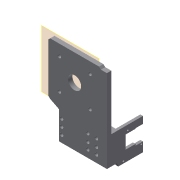
# Autodesk Inventor part: 10_Adapter_Laser_XY_left
Saved by Autodesk Inventor 2019 (Build 230136000, 136)
## iProperties
Created: 2019-05-02
Part Number: 10_Adapter_Laser_XY_left
Material: Generic
Document SubType Name: Modeling
Designer: diederichbenedict
Density: 1 g/cm^3
Appearance: Default
Author: diederichbenedict
Autodesk Inventor part; units mm, degrees
ref_plane "YZ Plane" through (0, 0, 0) normal (1, 0, 0) x (0, 1, 0)
ref_plane "XZ Plane" through (0, 0, 0) normal (0, 1, 0) x (-1, 0, 0)
ref_plane "XY Plane" through (0, 0, 0) normal (0, 0, 1) x (1, 0, 0)
ref_plane "Work Plane1" through (-10, 0, 0) normal (0, 0, 1) x (1, 0, 0)
sketch "Sketch1" plane through (-10, 0, 0) normal (0, 0, 1) x (1, 0, 0)
  line L0 (38, 30) -> (40, 28) construction
  line L1 (38, 30) -> (-18, 30) construction
  line L2 (-20, 28) -> (-18, 30) construction
  line L3 (-20, 28) -> (-20, -28) construction
  line L4 (-18, -30) -> (-20, -28) construction
  line L5 (-18, -30) -> (38, -30) construction
  line L6 (40, -28) -> (38, -30) construction
  line L7 (40, -28) -> (40, 28) construction
  circle A0 centre (-7.5, 17.5) radius 1.95 construction
  circle A1 centre (-7.5, -17.5) radius 1.95 construction
  circle A2 centre (27.5, -17.5) radius 1.95 construction
  circle A3 centre (27.5, 17.5) radius 1.95 construction
  circle A4 centre (10, 0) radius 7.5 construction
  circle A5 centre (-5, -51) radius 1 construction
  circle A6 centre (25, -58.5) radius 1 construction
  circle A7 centre (25, -42.5) radius 1.0474 construction
  circle A8 centre (35, -42.5) radius 1 construction
  circle A9 centre (35, -51) radius 1 construction
  circle A10 centre (35, -58.5) radius 1 construction
  circle A11 centre (25, -51) radius 1 construction
  circle A12 centre (-5, -59) radius 1 construction
  circle A13 centre (-5, -43) radius 1 construction
  line L8 (-8, -67) -> (-8, -35) construction
  line L9 (-8, -67) -> (40, -67) construction
  line L10 (40, -35) -> (40, -67) construction
  line L11 (-8, -35) -> (40, -35) construction
  line L12 (38, 30) -> (40, 28)
  line L13 (38, 30) -> (-18, 30)
  line L14 (-20, 28) -> (-18, 30)
  line L15 (-20, 28) -> (-20, -28)
  line L16 (-18, -30) -> (-20, -28)
  line L17 (-18, -30) -> (38, -30)
  line L18 (40, -28) -> (38, -30)
  line L19 (40, -28) -> (40, 28)
  circle A14 centre (-7.5, 17.5) radius 1.95
  circle A15 centre (-7.5, -17.5) radius 1.95
  circle A16 centre (27.5, -17.5) radius 1.95
  circle A17 centre (27.5, 17.5) radius 1.95
  circle A18 centre (10, 0) radius 7.5
  line L20 (-8, -35) -> (40, -35)
  line L21 (-8, -67) -> (-8, -35)
  line L22 (-8, -67) -> (40, -67)
  line L23 (40, -35) -> (40, -67)
  line L24 (-18, -30) -> (-8, -35)
  line L25 (40, -35) -> (40, -28)
  line L26 (40, -67) -> (47, -67)
  line L27 (47, -67) -> (47, -35)
  line L28 (47, -35) -> (40, -35)
  line L29 (40, -35) -> (40, -67)
  line L30 (40, -35) -> (47, -35)
  line L31 (47, -35) -> (47, -25)
  line L32 (47, -25) -> (40, -25)
  line L33 (40, -25) -> (40, -35)
  circle A19 centre (-5, -43) radius 1.5
  circle A20 centre (-5, -51) radius 1.5
  circle A21 centre (-5, -59) radius 1.5
  circle A22 centre (25, -42.5) radius 1.5
  circle A23 centre (25, -51) radius 1.5
  circle A24 centre (25, -58.5) radius 1.5
  circle A25 centre (35, -42.5) radius 1.5
  circle A26 centre (35, -51) radius 1.5
  circle A27 centre (35, -58.5) radius 1.5
  point P0 (10, 0)
extrude "Extrusion1" add sketch "Sketch1" along normal blind 5 contours L12 L19 L18 L17 L16 L15 L14 L13 | L25 L20 L24 L17 L18
sketch "Sketch2" plane through (30, -35, 0) normal (1, 0, 0) x (0, 0, -1)
  line L0 (0, 0) -> (0, 63) projected
  line L1 (0, 63) -> (-5, 63) projected
  line L2 (-5, 0) -> (-5, 63) projected
  line L3 (0, 0) -> (-5, 0) projected
  circle A0 centre (24, -16) radius 6 projected
  line L4 (8, -32) -> (40, -32) projected
  line L5 (40, -32) -> (40, 0) projected
  line L6 (40, 0) -> (8, 0) projected
  line L7 (8, 0) -> (8, -32) projected
  line L8 (8, -32) -> (5, -32)
  line L9 (5, -32) -> (5, 0)
  line L10 (5, 0) -> (8, 0)
  line L11 (8, 0) -> (8, -32)
  line L12 (5, 0) -> (-5, 12.3524)
  line L13 (0, 0) -> (-5, 0) projected
  line L14 (5, 0) -> (-5, 0)
  line L15 (-5, 0) -> (-5, 12.3524)
  point P0 (0, 35)
  dimension "d11" = 3
  constraints: 14 end point, 2 parallel, 2 perpendicular, 1 collinear, 1 horizontal, 1 point on line
  measures "d11" distance of L9.end L10.end
ref_plane "Work Plane2" through (-18, -67, -25) normal (-1, 0, 0) x (0, 0, 1)
extrude "Extrusion2" add sketch "Sketch2" against normal up to surface (48 mm away) contours L10 L7 L8 L9
sketch "Sketch4" plane through (30, -35, 0) normal (1, 0, 0) x (0, 0, -1)
  line L0 (0, 63) -> (-5, 63) projected
  line L1 (0, 0) -> (-5, 0) projected
  line L2 (-5, 0) -> (-5, 63) projected
  line L3 (0, 0) -> (0, 63) projected
  point P0 (0, 35)
ref_plane "Work Plane3" through (37, -80.7499, -30.1921) normal (-1, 0, 0) x (0, -0.417504, 0.9086751)
extrude "Extrusion4" add sketch "Sketch4" along normal up to surface (7 mm away)
sketch "Sketch5" plane through (37, -35, 0) normal (1, 0, 0) x (0, 0, -1)
  line L0 (0, 0) -> (-5, 0) construction
  line L1 (8, 0) -> (8, -32) construction
  circle A0 centre (14, -33.5) radius 1 construction
  circle A1 centre (34, -33.5) radius 1 construction
  circle A2 centre (19, -5.5) radius 1 construction
  line L2 (21.4305, -36) -> (8, -36) construction
  line L3 (-5, 0) -> (0, 0) projected
  line L4 (-5, 0) -> (8, -36)
  line L5 (8, -36) -> (36.2413, -36)
  line L6 (36.2413, -36) -> (36.2413, -25.2619)
  line L7 (36.2413, -25.2619) -> (27.7239, -25.2619)
  line L8 (27.7239, -25.2619) -> (27.7239, 0)
  line L9 (27.7239, 0) -> (0, 0)
  line L10 (0, 0) -> (-5, 0)
  circle A3 centre (24, -16) radius 2.6486 construction
  line L11 (31.5, -8.5) -> (16.5, -8.5)
  line L12 (16.5, -8.5) -> (16.5, -23.5)
  line L13 (16.5, -23.5) -> (31.5, -23.5)
  line L14 (31.5, -23.5) -> (31.5, -8.5)
  line L15 (31.5, -8.5) -> (16.5, -23.5) construction
  line L16 (16.5, -8.5) -> (31.5, -23.5) construction
  circle A4 centre (34.5, -27) radius 1 construction
  line L17 (27.7239, 0) -> (36.2413, 0)
  line L18 (36.2413, 0) -> (36.2413, -7.9172)
  line L19 (36.2413, -7.9172) -> (27.7239, -7.9172)
  line L20 (27.7239, -7.9172) -> (27.7239, 0)
  point P0 (0, 35)
  point P1 (27.7239, -23.5)
  point P2 (27.7239, -8.5)
  dimension "d38" = 15
  dimension "d39" = 15
  constraints: 34 end point, 6 perpendicular, 5 equal length, 4 point on line, 3 horizontal, 2 midpoint
  measures "d38" distance of L13.end L12.end
  measures "d39" distance of L12.end L11.end
extrude "Extrusion5" add sketch "Sketch5" against normal blind 3 contours L3 L9 L8 L11 L12 L13 L7 L6 L5 L4 | L17 L18 L19 L8
ref_plane "Work Plane4" through (37, -71, -27) normal (0, -1, 0) x (1, 0, 0)
sketch "Sketch8" plane through (37, 28, 5) normal (1, 0, 0) x (0, 0, -1)
  circle A0 centre (19, -96.5) radius 1 projected
  line L0 (16, -99) -> (41.7, -99) projected
  circle A1 centre (39.5, -90) radius 1 projected
  circle A2 centre (24, -68.5) radius 1 projected
  point P0 (5, -28)
extrude "Extrusion8" cut sketch "Sketch8" against normal through all
sketch "Sketch9" plane through (-18, -67, -5) normal (-1, 0, 0) x (0, 0, 1)
  line L0 (-3, 0) -> (0, 0) construction
  line L1 (0, 0) -> (0, 32) construction
  line L2 (-3, 0) -> (-3, 32) construction
  line L3 (0, 32) -> (-3, 32) construction
  line L4 (-3, 0) -> (10, 32) construction
  line L5 (5, 32) -> (10, 32) construction
  line L6 (10, 32) -> (0, 32) construction
  line L7 (0, 32) -> (10, 32)
  line L8 (10, 32) -> (10, 0)
  line L9 (10, 0) -> (0, 0)
  line L10 (0, 0) -> (0, 32)
  line L11 (-3, 32) -> (0, 32)
  line L12 (0, 32) -> (0, 0)
  line L13 (0, 0) -> (-3, 0)
  line L14 (-3, 0) -> (-3, 32)
  point P0 (5, 67)
  constraints: 18 end point, 4 parallel, 3 horizontal, 2 perpendicular
extrude "Extrusion9" add sketch "Sketch9" against normal up to surface (55 mm away)
sketch "Sketch10" plane through (-18, -59.6154, 5) normal (0, 0, 1) x (-1, 0, 0)
  circle A0 centre (-3, -8.6154) radius 1 construction
  circle A1 centre (-3, -16.6154) radius 1 construction
  circle A2 centre (-3, -0.6154) radius 1 construction
  circle A3 centre (-33, -8.6154) radius 1 construction
  circle A4 centre (-33, -1.1154) radius 1 construction
  circle A5 centre (-33, -17.1154) radius 1.0474 construction
  circle A6 centre (-43, -17.1154) radius 1 construction
  line L0 (-43, -14.6154) -> (-43, -2.6154) construction
  circle A7 centre (-43, -8.6154) radius 1 construction
  circle A8 centre (-43, -1.1154) radius 1 construction
  circle A9 centre (-3, -16.6154) radius 2
  circle A10 centre (-33, -17.1154) radius 2
  circle A11 centre (-43, -17.1154) radius 2
  circle A12 centre (-43, -8.6154) radius 2
  circle A13 centre (-43, -1.1154) radius 2
  circle A14 centre (-33, -8.6154) radius 2
  circle A15 centre (-33, -1.1154) radius 2
  circle A16 centre (-3, -8.6154) radius 2
  circle A17 centre (-3, -0.6154) radius 2
  point P0 (-18, -59.6154)
  dimension "d40" = 4
  dimension "d41" = 4
  dimension "d42" = 4
  dimension "d43" = 4
  dimension "d44" = 4
  dimension "d45" = 4
  dimension "d46" = 4
  dimension "d47" = 4
  dimension "d48" = 4
  constraints: 9 centre point, 9 coincident
  measures "d40" diameter of A9
  measures "d41" diameter of A10
  measures "d42" diameter of A11
  measures "d43" diameter of A12
  measures "d44" diameter of A13
  measures "d45" diameter of A14
  measures "d46" diameter of A15
  measures "d47" diameter of A16
  measures "d48" diameter of A17
extrude "Extrusion10" cut sketch "Sketch10" along normal through all both and the other way through all
body "Solid1"
